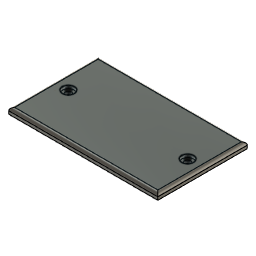
tundra_base_cover (Autodesk Fusion 360 design; units mm, degrees)
Autodesk Fusion 360 part; units mm, degrees
sketch "Sketch1" plane through (0, 0, 0) normal (0, 0, 1) x (1, 0, 0)
  line L0 (0, 0) -> (50, 0)
  line L1 (50, 0) -> (50, 30)
  line L2 (50, 30) -> (0, 30)
  line L3 (0, 30) -> (0, 0)
  dimension "d1" = 50
  dimension "d2" = 30
  constraint horizontal L0
  constraint vertical L1
  constraint horizontal L2
  constraint vertical L3
  constraint coincident L0.start L3.end
  measures "d1" distance of L0.start L0.end
  measures "d2" distance of L0.start L2.end
extrude "Extrude1" add sketch "Sketch1" along normal blind 2
fillet "Fillet1" radius 1 1 faces at (16.6667, 20, 2)
sketch "Sketch2" plane through (0, 0, 2) normal (0, 0, 1) x (-1, 0, 0)
  line L0 (-49, -1) -> (-49, -29)
  line L1 (-49, -29) -> (-1, -29)
  line L2 (-1, -29) -> (-1, -1)
  line L3 (-1, -1) -> (-49, -1)
  circle A0 centre (-5, -15) radius 1
  circle A1 centre (-45, -15) radius 1
  line L4 (0, -30) -> (0, 0)
  line L5 (-50, -30) -> (0, -30)
  dimension "d7" = 2
  dimension "d8" = 2
  dimension "d9" = 40
  dimension "d10" = 5
  dimension "d11" = 15
  measures "d7" diameter of A1
  measures "d8" diameter of A0
  measures "d9" distance of A0.centre A1.centre
  measures "d10" distance of A0.centre L4
  measures "d11" distance of A0.centre L5
extrude "Extrude2" cut sketch "Sketch2" against normal blind 1 contours A0 | A1
sketch "Sketch3" plane through (0, 0, 2) normal (0, 0, 1) x (-1, 0, 0)
  circle A0 centre (-45, -15) radius 1
  circle A1 centre (-5, -15) radius 1
  line L0 (-49, -1) -> (-49, -29)
  line L1 (-49, -29) -> (-1, -29)
  line L2 (-1, -29) -> (-1, -1)
  line L3 (-1, -1) -> (-49, -1)
  circle A2 centre (-5, -15) radius 2
  circle A3 centre (-45, -15) radius 2
  dimension "d14" = 4
  dimension "d15" = 4
  constraint concentric A1 A2
  constraint concentric A0 A3
  measures "d14" diameter of A2
  measures "d15" diameter of A3
extrude "Extrude4" cut sketch "Sketch3" against normal blind 11 contours A0 | A1
extrude "Extrude5" cut sketch "Sketch3" against normal blind 1 contours A2 | A3
extrude "Extrude3" [suppressed]
